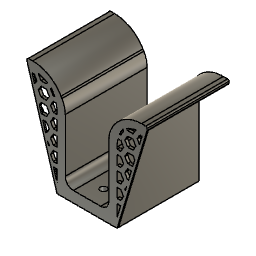
Antriebsabdeckung v4 (Autodesk Fusion 360 design; units mm, degrees)
Autodesk Fusion 360 part; units mm, degrees
note: some values were not read from the file. Set by a fixed rule: which sketch regions a step uses.
sketch "Skizze1" plane through (0, 0, 0) normal (0, 0, 1) x (1, 0, 0)
  line L0 (-250, 150) -> (-30, 150)
  line L1 (-30, 150) -> (-30, -150)
  line L2 (-30, -150) -> (-250, -150)
  line L3 (-250, -150) -> (-250, 150)
  dimension "d1" = 220
  dimension "d2" = 300
  constraint horizontal L0
  constraint vertical L1
  constraint horizontal L2
  constraint vertical L3
  measures "d1" distance of L0.start L0.end
  measures "d2" distance of L0.start L2.end
sketch "Skizze1 (2)" plane through (0, 0, 0) normal (0, 0, 1) x (1, 0, 0) in component "Component'"
  line L0 (0, 30) -> (22, 30)
  line L1 (22, 30) -> (22, 0)
  line L2 (22, 0) -> (0, 0)
  line L3 (0, 0) -> (0, 30)
  dimension "d5" = 22
  dimension "d6" = 30
  constraint horizontal L0
  constraint vertical L1
  constraint horizontal L2
  constraint vertical L3
  constraint coincident L2.end L3.start
  measures "d5" distance of L0.start L0.end
  measures "d6" distance of L0.start L2.end
extrude "Extrusion1" add sketch "Skizze1 (2)" along normal blind 4 in component "Component'"
sketch "Skizze2" plane through (0, 0, 0) normal (0, 0, 1) x (1, 0, 0) in component "Component'"
  line L0 (0, 30) -> (3, 30)
  line L1 (3, 30) -> (3, 0)
  line L2 (3, 0) -> (0, 0)
  line L3 (0, 0) -> (0, 30)
  line L4 (19, 30) -> (22, 30)
  line L5 (22, 30) -> (22, 0)
  line L6 (22, 0) -> (19, 0)
  line L7 (19, 0) -> (19, 30)
  dimension "d9" = 3
  dimension "d10" = 30
  dimension "d11" = 3
  dimension "d12" = 30
  constraint horizontal L0
  constraint vertical L1
  constraint horizontal L2
  constraint vertical L3
  constraint coincident L2.end L3.start
  constraint horizontal L4
  constraint vertical L5
  constraint horizontal L6
  constraint vertical L7
  measures "d9" distance of L0.start L0.end
  measures "d10" distance of L0.start L2.end
  measures "d11" distance of L4.start L4.end
  measures "d12" distance of L4.start L6.end
extrude "Extrusion2" add sketch "Skizze2" along normal blind 29 in component "Component'"
fillet "Abrundung1" radius 3 1 edges at (3, 15, 4) in component "Component'"
fillet "Abrundung2" radius 3 1 edges at (19, 15, 4) in component "Component'"
sketch "Skizze3" plane through (0, 0, 0) normal (0, 1, 0) x (1, 0, 0) in component "Component'"
  line L0 (22, -29) -> (27, -37.6603)
  line L1 (22, -29) -> (29, -29) construction
  line L2 (27, -37.6603) -> (24, -37.6603)
  line L3 (24, -37.6603) -> (19, -29)
  line L4 (19, -29) -> (19, -28)
  line L5 (19, -28) -> (22, -28)
  line L6 (22, -28) -> (22, -29)
  line L7 (3, -28) -> (3, -29)
  line L8 (3, -28) -> (0, -28)
  line L9 (0, -28) -> (0, -29)
  line L10 (0, -29) -> (-5, -37.6603)
  line L11 (-5, -37.6603) -> (-2, -37.6603)
  line L12 (-2, -37.6603) -> (3, -29)
  dimension "d19" = 60
  dimension "d20" = 10
  dimension "d21" = 3
  dimension "d22" = 30
  dimension "d23" = 10
  dimension "d24" = 60
  dimension "d25" = 3
  constraint horizontal L1
  constraint horizontal L2
  constraint perpendicular L2 L4
  constraint perpendicular L4 L5
  constraint perpendicular L1 L6
  constraint perpendicular L5 L7
  constraint perpendicular L7 L8
  constraint perpendicular L8 L9
  measures "d19" angle of L0 L1
  measures "d20" distance of L0.start L0.end
  measures "d21" distance of L0.end L2.end
  measures "d22" angle of L9 L10
  measures "d23" distance of L9.end L10.end
  measures "d24" angle of L10 L11
  measures "d25" distance of L10.end L11.end
extrude "Extrusion3" add sketch "Skizze3" along normal blind 30 in component "Component'"
fillet "Abrundung3" radius 12 1 edges at (22, 15, 29) in component "Component'"
fillet "Abrundung4" radius 12 1 edges at (0, 15, 29) in component "Component'"
fillet "Abrundung5" radius 9 2 edges at (19, 15, 29) (3, 15, 29) in component "Component'"
sketch "Skizze4" plane through (0, 0, 0) normal (0, 1, 0) x (1, 0, 0) in component "Component'"
  line L0 (27, -37.6603) -> (33, -37.6603)
  line L1 (33, -37.6603) -> (33, -36.1603)
  line L2 (27, -37.6603) -> (24.3973, -33.167)
  line L3 (24.3973, -33.167) -> (33, -36.1603)
  line L4 (0, -2.5) -> (22, -2.5)
  line L5 (11, -2.5) -> (11, -47.5)
  point P0 (27, -37.6603)
  dimension "d34" = 6
  dimension "d35" = 1.5
  dimension "d39" = 45
  constraint horizontal L0
  constraint coincident P0 L0.start
  constraint vertical L1
  constraint horizontal L4
  constraint vertical L5
  constraint midpoint L4 L5.start
  measures "d34" distance of P0 L0.end
  measures "d35" distance of L0.end L1.end
  measures "d39" distance of L5.start L5.end
extrude "Extrusion4" add sketch "Skizze4" along normal blind 30 in component "Component'"
fillet "Abrundung6" radius 5 1 edges at (24.4079, 15, 33.1707) in component "Component'"
fillet "Abrundung7" radius 12 1 edges at (24, 15, 37.6603) in component "Component'"
fillet "Abrundung8" radius 0.5 1 edges at (33, 15, 37.6603) in component "Component'"
fillet "Abrundung9" radius 0.5 1 edges at (33, 15, 36.1603) in component "Component'"
sketch "Skizze5" plane through (0, 0, 0) normal (0, -1, 0) x (1, 0, 0) in component "Component'"
  arc A0 (32.6643, 36.0435) -> (33, 36.5157) centre (32.5, 36.5157) ccw
  line L0 (33, 36.5157) -> (33, 37.1603)
  arc A1 (33, 37.1603) -> (32.5, 37.6603) centre (32.5, 37.1603) ccw
  line L1 (32.5, 37.6603) -> (30.9282, 37.6603)
  arc A2 (30.9282, 37.6603) -> (20.5359, 31.6603) centre (30.9282, 25.6603) ccw
  line L2 (20.5359, 31.6603) -> (20.2058, 31.0885)
  arc A3 (20.2058, 31.0885) -> (19, 26.5885) centre (28, 26.5885) ccw
  line L3 (19, 26.5885) -> (19, 7)
  arc A4 (16, 4) -> (19, 7) centre (16, 7) ccw
  line L4 (16, 4) -> (6, 4)
  arc A5 (3, 7) -> (6, 4) centre (6, 7) ccw
  line L5 (3, 7) -> (3, 26.5885)
  arc A6 (3, 26.5885) -> (1.7942, 31.0885) centre (-6, 26.5885) ccw
  line L6 (1.7942, 31.0885) -> (-2, 37.6603)
  line L7 (-2, 37.6603) -> (-5, 37.6603)
  line L8 (-5, 37.6603) -> (-1.6077, 31.7846)
  arc A7 (0, 25.7846) -> (-1.6077, 31.7846) centre (-12, 25.7846) ccw
  line L9 (0, 25.7846) -> (0, 0)
  line L10 (0, 0) -> (22, 0)
  line L11 (22, 0) -> (22, 25.7846)
  arc A8 (23.3965, 31.403) -> (22, 25.7846) centre (34, 25.7846) ccw
  arc A9 (26.1715, 33.7843) -> (23.3965, 31.403) centre (27.8146, 29.062) ccw
  line L12 (26.1715, 33.7843) -> (32.6643, 36.0435)
  line L13 (-5, 37.6603) -> (-11, 37.6603)
  line L14 (-11, 37.6603) -> (-11, 36.1603)
  line L15 (-11, 36.1603) -> (-2.3934, 33.1455)
  line L16 (-5, 37.6603) -> (-4.6132, 37.6603)
  line L17 (-4.6132, 37.6603) -> (-1.8556, 32.8839)
  line L18 (-1.8556, 32.8839) -> (-2.3934, 33.1455)
  dimension "d50" = 6
  dimension "d51" = 1.5
  constraint coincident L7.end L8.start
  constraint parallel L7 L13
  constraint perpendicular L13 L14
  constraint coincident L8 L15.end
  constraint coincident L7 L16.end
  constraint parallel L8 L17
  measures "d50" distance of L7.end L13.end
  measures "d51" distance of L13.end L14.end
extrude "Extrusion5" add sketch "Skizze5" against normal blind 30 contours L8 L13 L14 L15 in component "Component'"
fillet "Abrundung10" radius 12 1 edges at (-2, 15, 37.6603) in component "Component'"
fillet "Abrundung11" radius 0.5 1 edges at (-11, 15, 37.6603) in component "Component'"
fillet "Abrundung12" radius 0.5 1 edges at (-11, 15, 36.1603) in component "Component'"
fillet "Abrundung13" radius 5 1 edges at (-2.3934, 15, 33.1455) in component "Component'"
sketch "Skizze6" plane through (0, 0, 0) normal (0, 1, 0) x (1, 0, 0) in component "Component'"
  line L0 (0, 0) -> (22, 0)
  line L1 (11, 0) -> (11, -40)
  line L2 (0, 0) -> (-11, -36.5149)
  line L3 (0, 0) -> (-11, -36.5149)
  line L4 (-11, -36.5149) -> (-10.0425, -36.8033)
  line L5 (-10.0425, -36.8033) -> (0.9575, -0.2884)
  line L6 (0.9575, -0.2884) -> (0, 0)
  point P0 (-11, -36.5149)
  dimension "d63" = 22
  dimension "d64" = 40
  dimension "d65" = 1
  constraint coincident L0.start L2.start
  constraint horizontal L0
  constraint midpoint L0 L1.start
  constraint perpendicular L0 L1
  constraint coincident P0 L2.end
  constraint perpendicular L3 L4
  constraint parallel L3 L5
  constraint parallel L4 L6
  measures "d63" distance of L0.start L0.end
  measures "d64" distance of L1.start L1.end
  measures "d65" distance of L0.start L5.end
sketch "Skizze7" plane through (-1.5503, 0, 28.8306) normal (0, 1, 0) x (1, 0, 0) in component "Component'"
sketch "Skizze8" plane through (0, 0, 0) normal (0, 1, 0) x (1, 0, 0) in component "Component'"
sketch "Skizze9" plane through (0, 0, 0) normal (0, 1, 0) x (1, 0, 0) in component "Component'"
  line L0 (0, 0) -> (22, 0)
  line L1 (22, 0) -> (33, -36.5157)
  line L2 (22, 0) -> (33, -36.5157)
  line L3 (33, -36.5157) -> (32.0425, -36.8041)
  line L4 (32.0425, -36.8041) -> (21.0425, -0.2884)
  line L5 (21.0425, -0.2884) -> (22, 0)
  point P0 (33, -36.5157)
  dimension "d98" = 22
  dimension "d99" = 1
  constraint coincident L0.start origin
  constraint horizontal L0
  constraint coincident P0 L1.end
  constraint perpendicular L2 L3
  constraint parallel L2 L4
  constraint parallel L3 L5
  constraint parallel L1 L2
  measures "d98" distance of L0.start L0.end
  measures "d99" distance of L0.end L4.end
extrude "Extrusion6" add sketch "Skizze9" sketch "Skizze6" along normal blind 1 of sketch 2 in component "Component'"
fillet "Abrundung14" radius 0.5 1 edges at (-4.8565, 1, 19.5882) in component "Component'"
fillet "Abrundung15" radius 0.5 1 edges at (-5.4584, 1, 18.1194) in component "Component'"
fillet "Abrundung16" radius 0.5 1 edges at (27.4584, 1, 18.1198) in component "Component'"
fillet "Abrundung17" radius 0.5 1 edges at (26.8569, 1, 19.5898) in component "Component'"
sketch "Skizze10" plane through (0, 0, 0) normal (0, 1, 0) x (1, 0, 0) in component "Component'"
  line L0 (-1.3615, -7.8038) -> (0.6385, -7.804)
  line L1 (0.6389, -4.3399) -> (-0.6992, -4.3399)
  line L2 (-1.6032, -7.3682) -> (-1.3615, -7.8038)
  line L3 (-1.3615, -7.8038) -> (-0.3615, -7.8039) construction
  line L4 (-2.3613, -11.2682) -> (-1.3615, -9.536)
  line L5 (-1.3615, -9.536) -> (-0.3615, -9.5359) construction
  line L6 (-1.3615, -9.536) -> (0.6385, -9.5358)
  line L7 (-1.3611, -13.0001) -> (-2.3613, -11.2682)
  line L8 (0.6389, -12.9999) -> (-1.3611, -13.0001)
  line L9 (-1.3615, -9.536) -> (-0.3615, -9.5359) construction
  line L10 (-2.3613, -11.2682) -> (-1.3615, -9.536)
  line L11 (-1.3615, -9.536) -> (0.6385, -9.5358)
  line L12 (-1.3611, -13.0001) -> (-2.3613, -11.2682)
  line L13 (0.6389, -12.9999) -> (-1.3611, -13.0001)
  line L14 (-1.3613, -33.7846) -> (-3.4883, -33.7846) construction
  line L15 (-1.3613, -30.3205) -> (-2.3613, -32.0526)
  line L16 (-2.3613, -32.0526) -> (-1.3613, -33.7846)
  line L17 (0.6387, -30.3205) -> (-1.3613, -30.3205)
  line L18 (-7.3878, -32.0984) -> (-8.5461, -30.1296)
  line L19 (-9.6744, -33.7729) -> (-8.3545, -33.7729)
  line L20 (-8.3545, -33.7729) -> (-7.3878, -32.0984)
  line L21 (-1.3613, -18.1962) -> (0.6387, -18.1962)
  line L22 (-1.3613, -14.7321) -> (-2.3613, -16.4641)
  line L23 (-2.3613, -16.4641) -> (-1.3613, -18.1962)
  line L24 (0.6387, -14.7321) -> (-1.3613, -14.7321)
  line L25 (-1.3613, -28.5885) -> (0.6387, -28.5885)
  line L26 (-1.3613, -25.1244) -> (-2.3613, -26.8564)
  line L27 (-2.3613, -26.8564) -> (-1.3613, -28.5885)
  line L28 (0.6387, -25.1244) -> (-1.3613, -25.1244)
  line L29 (-2.8613, -34.6506) -> (-3.8613, -32.9186)
  line L30 (-5.8613, -32.9186) -> (-6.8613, -34.6506)
  line L31 (-6.8613, -34.6506) -> (-5.8613, -36.3827)
  line L32 (-3.8613, -32.9186) -> (-5.8613, -32.9186)
  line L33 (-2.8613, -29.4545) -> (-3.8613, -27.7224)
  line L34 (-5.8613, -31.1865) -> (-3.8613, -31.1865)
  line L35 (-5.8613, -27.7224) -> (-6.8613, -29.4545)
  line L36 (-3.8613, -31.1865) -> (-2.8613, -29.4545)
  line L37 (-6.8613, -29.4545) -> (-5.8613, -31.1865)
  line L38 (-3.8613, -27.7224) -> (-5.8613, -27.7224)
  line L39 (-2.8613, -19.0622) -> (-3.8684, -17.3179)
  line L40 (-5.6515, -20.7821) -> (-3.8543, -20.7821)
  line L41 (-3.8543, -20.7821) -> (-2.8613, -19.0622)
  line L42 (-3.8684, -17.3179) -> (-4.5785, -17.3174)
  line L43 (-1.3613, -23.3923) -> (0.6387, -23.3923)
  line L44 (-1.3613, -19.9282) -> (-2.3613, -21.6603)
  line L45 (-2.3613, -21.6603) -> (-1.3613, -23.3923)
  line L46 (0.6387, -19.9282) -> (-1.3613, -19.9282)
  line L47 (0, 0) -> (22, 0)
  line L48 (11, 0) -> (11, -45)
  line L49 (1.1387, -3.4737) -> (-0.4406, -3.4736)
  line L50 (22, -3.467) -> (22, -25.7846)
  line L51 (0.6387, -25.1244) -> (0.6387, -28.5885)
  line L52 (0.6387, -23.3923) -> (0.6387, -19.9282)
  line L53 (0.6387, -14.7321) -> (0.6387, -18.1962)
  line L54 (0.6387, -30.3205) -> (-1.3613, -33.7846)
  line L55 (-2.8613, -34.6506) -> (-5.8613, -36.3827)
  line L56 (0.6389, -4.3399) -> (0.6385, -7.804)
  line L57 (1.1387, -3.4737) -> (1.1387, -8.6699)
  line L58 (0.6385, -9.5358) -> (0.6389, -12.9999)
  line L59 (1.1387, -8.6699) -> (1.1387, -13.866)
  line L60 (1.1387, -13.866) -> (1.1387, -19.0622)
  line L61 (1.1387, -19.0622) -> (1.1387, -24.2583)
  line L62 (1.1387, -24.2583) -> (1.1387, -29.4545)
  line L63 (1.1387, -29.4545) -> (0.6387, -31.9352)
  line L64 (0.6387, -31.9352) -> (-0.8065, -33.9794)
  line L65 (-0.8065, -33.9794) -> (-1.8613, -34.6506)
  line L66 (-6.4159, -37.1736) -> (-1.8613, -34.6506)
  line L67 (-5.8613, -25.9904) -> (-3.8613, -25.9904)
  line L68 (-3.8613, -22.5263) -> (-5.8613, -22.5263)
  line L69 (-6.8613, -24.2583) -> (-5.8613, -25.9904)
  line L70 (-5.8613, -22.5263) -> (-6.8613, -24.2583)
  line L71 (-2.8613, -24.2583) -> (-3.8613, -22.5263)
  line L72 (-3.8613, -25.9904) -> (-2.8613, -24.2583)
  line L73 (-2.8613, -13.866) -> (-3.3053, -13.07)
  line L74 (-3.8613, -15.5981) -> (-2.8613, -13.866)
  line L75 (-4.06, -15.5981) -> (-3.8613, -15.5981)
  line L76 (-10.3496, -35.9533) -> (-8.3613, -35.5167)
  line L77 (-8.3613, -35.5167) -> (-7.3613, -37.2487)
  line L78 (-6.4159, -37.1736) -> (-7.3613, -37.2487)
  line L79 (-10.3496, -35.9533) -> (-4.4333, -16.8484)
  line L80 (-4.4333, -16.8484) -> (-0.4406, -3.4736)
  line L81 (-1.6032, -7.3682) -> (-1.9229, -8.4393)
  line L82 (-0.4406, -3.4736) -> (-0.6992, -4.3399)
  line L83 (-1.6032, -7.3682) -> (-1.9229, -8.4393)
  line L84 (-5.6515, -20.7821) -> (-7.4138, -26.5466)
  line L85 (27.8613, -22.5263) -> (28.8613, -24.2583)
  line L86 (21.3611, -12.9999) -> (23.3611, -13.0001)
  line L87 (23.3611, -13.0001) -> (24.3613, -11.2682)
  line L88 (25.8613, -15.5981) -> (24.8613, -13.866)
  line L89 (20.8613, -13.866) -> (20.8613, -19.0622)
  line L90 (24.8613, -13.866) -> (25.3053, -13.07)
  line L91 (23.3611, -13.0001) -> (24.3613, -11.2682)
  line L92 (20.8613, -3.4737) -> (22.4406, -3.4736)
  line L93 (24.3613, -16.4641) -> (23.3613, -18.1962)
  line L94 (23.3613, -14.7321) -> (24.3613, -16.4641)
  line L95 (23.3615, -9.536) -> (21.3615, -9.5358)
  line L96 (21.3611, -12.9999) -> (23.3611, -13.0001)
  line L97 (21.3613, -14.7321) -> (21.3613, -18.1962)
  line L98 (23.6032, -7.3682) -> (23.3615, -7.8038)
  line L99 (21.3613, -14.7321) -> (23.3613, -14.7321)
  line L100 (22.4406, -3.4736) -> (22.6992, -4.3399)
  line L101 (26.06, -15.5981) -> (25.8613, -15.5981)
  line L102 (20.8613, -3.4737) -> (20.8613, -8.6699)
  line L103 (31.6744, -33.7729) -> (30.3545, -33.7729)
  line L104 (23.3613, -30.3205) -> (24.3613, -32.0526)
  line L105 (29.3878, -32.0984) -> (30.5461, -30.1296)
  line L106 (21.3613, -31.9352) -> (22.8065, -33.9794)
  line L107 (21.3613, -30.3205) -> (23.3613, -30.3205)
  line L108 (27.8613, -31.1865) -> (25.8613, -31.1865)
  line L109 (28.8613, -24.2583) -> (27.8613, -25.9904)
  line L110 (25.8684, -17.3179) -> (26.5785, -17.3174)
  line L111 (27.8613, -32.9186) -> (28.8613, -34.6506)
  line L112 (21.3613, -25.1244) -> (21.3613, -28.5885)
  line L113 (30.3545, -33.7729) -> (29.3878, -32.0984)
  line L114 (27.6515, -20.7821) -> (25.8543, -20.7821)
  line L115 (25.8613, -27.7224) -> (27.8613, -27.7224)
  line L116 (24.3613, -26.8564) -> (23.3613, -28.5885)
  line L117 (21.3613, -30.3205) -> (23.3613, -33.7846)
  line L118 (25.8613, -32.9186) -> (27.8613, -32.9186)
  line L119 (20.8613, -24.2583) -> (20.8613, -29.4545)
  line L120 (25.8613, -22.5263) -> (27.8613, -22.5263)
  line L121 (28.8613, -29.4545) -> (27.8613, -31.1865)
  line L122 (27.8613, -27.7224) -> (28.8613, -29.4545)
  line L123 (23.3613, -28.5885) -> (21.3613, -28.5885)
  line L124 (24.3613, -32.0526) -> (23.3613, -33.7846)
  line L125 (28.4159, -37.1736) -> (29.3613, -37.2487)
  line L126 (24.8613, -29.4545) -> (25.8613, -27.7224)
  line L127 (25.8543, -20.7821) -> (24.8613, -19.0622)
  line L128 (20.8613, -29.4545) -> (21.3613, -31.9352)
  line L129 (23.3613, -23.3923) -> (21.3613, -23.3923)
  line L130 (24.8613, -19.0622) -> (25.8684, -17.3179)
  line L131 (25.8613, -25.9904) -> (24.8613, -24.2583)
  line L132 (23.3613, -18.1962) -> (21.3613, -18.1962)
  line L133 (23.3613, -25.1244) -> (24.3613, -26.8564)
  line L134 (27.6515, -20.7821) -> (29.4138, -26.5466)
  line L135 (30.3613, -35.5167) -> (29.3613, -37.2487)
  line L136 (23.3613, -33.7846) -> (25.4883, -33.7846) construction
  line L137 (24.8613, -34.6506) -> (25.8613, -32.9186)
  line L138 (22.8065, -33.9794) -> (23.8613, -34.6506)
  line L139 (24.3613, -21.6603) -> (23.3613, -23.3923)
  line L140 (20.8613, -19.0622) -> (20.8613, -24.2583)
  line L141 (21.3613, -23.3923) -> (21.3613, -19.9282)
  line L142 (27.8613, -25.9904) -> (25.8613, -25.9904)
  line L143 (24.8613, -24.2583) -> (25.8613, -22.5263)
  line L144 (32.3496, -35.9533) -> (30.3613, -35.5167)
  line L145 (28.4159, -37.1736) -> (23.8613, -34.6506)
  line L146 (26.4333, -16.8484) -> (22.4406, -3.4736)
  line L147 (21.3613, -19.9282) -> (23.3613, -19.9282)
  line L148 (21.3615, -9.5358) -> (21.3611, -12.9999)
  line L149 (24.8613, -34.6506) -> (27.8613, -36.3827)
  line L150 (21.3613, -25.1244) -> (23.3613, -25.1244)
  line L151 (28.8613, -34.6506) -> (27.8613, -36.3827)
  line L152 (25.8613, -31.1865) -> (24.8613, -29.4545)
  line L153 (24.3613, -11.2682) -> (23.3615, -9.536)
  line L154 (23.3613, -19.9282) -> (24.3613, -21.6603)
  line L155 (23.3615, -9.536) -> (22.3615, -9.5359) construction
  line L156 (23.3615, -9.536) -> (21.3615, -9.5358)
  line L157 (24.3613, -11.2682) -> (23.3615, -9.536)
  line L158 (23.6032, -7.3682) -> (23.9229, -8.4393)
  line L159 (23.3615, -7.8038) -> (21.3615, -7.804)
  line L160 (32.3496, -35.9533) -> (26.4333, -16.8484)
  line L161 (21.3611, -4.3399) -> (21.3615, -7.804)
  line L162 (21.3611, -4.3399) -> (22.6992, -4.3399)
  line L163 (23.3615, -7.8038) -> (22.3615, -7.8039) construction
  line L164 (23.6032, -7.3682) -> (23.9229, -8.4393)
  line L165 (20.8613, -8.6699) -> (20.8613, -13.866)
  line L166 (23.3615, -9.536) -> (22.3615, -9.5359) construction
  point P0 (1.1387, -8.6699)
  point P1 (-0.3613, -11.268)
  point P2 (-0.3613, -21.6603)
  point P3 (-4.8613, -19.0622)
  point P4 (-0.3613, -26.8564)
  point P5 (-4.8613, -29.4545)
  point P6 (-4.66, -23.9097)
  point P7 (-9.3613, -32.0526)
  point P8 (-4.8613, -34.6506)
  point P9 (-0.3613, -32.0526)
  point P10 (-9.3613, -37.2487)
  point P11 (-9.3613, -37.2487)
  point P12 (-0.3613, -32.0526)
  point P13 (-9.3613, -32.0526)
  point P14 (-0.3613, -16.4641)
  point P15 (-4.8613, -13.866)
  point P16 (-0.3613, -26.8564)
  point P17 (-4.8613, -34.6506)
  point P18 (-4.8613, -29.4545)
  point P19 (-4.66, -23.9097)
  point P20 (-4.8613, -19.0622)
  point P21 (-0.3613, -21.6603)
  point P22 (-4.8613, -24.2583)
  point P23 (-4.8613, -24.2583)
  point P24 (-4.8613, -13.866)
  point P25 (-4.8613, -13.866)
  point P26 (22.3613, -21.6603)
  point P27 (26.8613, -19.0622)
  point P28 (26.8613, -13.866)
  point P29 (26.8613, -19.0622)
  point P30 (20.8613, -8.6699)
  point P31 (26.8613, -13.866)
  point P32 (26.8613, -24.2583)
  point P33 (22.3613, -21.6603)
  point P34 (26.8613, -24.2583)
  point P35 (26.66, -23.9097)
  point P36 (26.66, -23.9097)
  point P37 (22.3613, -16.4641)
  point P38 (26.8613, -13.866)
  point P39 (22.3613, -26.8564)
  point P40 (26.8613, -34.6506)
  point P41 (26.8613, -29.4545)
  point P42 (22.3613, -32.0526)
  point P43 (22.3613, -11.268)
  point P44 (26.8613, -29.4545)
  point P45 (22.3613, -32.0526)
  point P46 (31.3613, -37.2487)
  point P47 (22.3613, -26.8564)
  point P48 (31.3613, -32.0526)
  point P49 (31.3613, -32.0526)
  point P50 (31.3613, -37.2487)
  point P51 (26.8613, -34.6506)
  dimension "d119" = 0
  dimension "d144" = 22
  dimension "d145" = 45
  dimension "d149" = 20
  constraint horizontal L14
  constraint coincident P11 P10
  constraint coincident P13 P7
  constraint coincident P17 P8
  constraint coincident P18 P5
  constraint coincident P19 P6
  constraint coincident P21 P2
  constraint coincident P12 P9
  constraint coincident P16 P4
  constraint coincident P20 P3
  constraint coincident L47.start origin
  constraint horizontal L47
  constraint vertical L48
  constraint midpoint L47 L48.start
  constraint perpendicular L25 L51
  constraint perpendicular L46 L52
  constraint perpendicular L31 L55
  constraint coincident P0 L57.end
  constraint coincident P23 P22
  constraint coincident P25 P24
  constraint coincident L1.end L80
  constraint horizontal L1
  constraint coincident L2.start L80
  constraint coincident L81.end L80
  constraint coincident L73.end L80
  constraint coincident L75.start L80
  constraint coincident L42.end L79
  constraint coincident L40.start L79
  constraint horizontal L40
  constraint horizontal L19
  constraint coincident L19.start L79
  constraint coincident L18.end L79
  constraint symmetric L49.start L48 L92.start
  constraint symmetric L81.end L48 L158.end
  constraint symmetric L0.start L48 L98.end
  constraint symmetric L0.end L48 L159.end
  constraint symmetric L1.start L48 L161.start
  constraint symmetric L1.end L48 L100.end
  constraint symmetric L2.start L48 L98.start
  constraint symmetric L3.end L48 L163.end
  constraint symmetric L7.start L48 L86.end
  constraint symmetric L4.start L48 L87.end
  constraint symmetric P0 L48 P30
  constraint symmetric L5.end L48 L155.end
  constraint symmetric L59.end L48 L89.start
  constraint symmetric L6.end L48 L95.end
  constraint symmetric L4.end L48 L95.start
  constraint symmetric L8.start L48 L86.start
  constraint symmetric P1 L48 P43
  constraint symmetric L60.end L48 L89.end
  constraint symmetric L61.end L48 L119.start
  constraint symmetric P21 L48 P33
  constraint symmetric P20 L48 P29
  constraint symmetric L62.end L48 L119.end
  constraint symmetric P16 L48 P47
  constraint symmetric P18 L48 P44
  constraint symmetric P19 L48 P36
  constraint symmetric P13 L48 P49
  constraint symmetric L65.end L48 L138.end
  constraint symmetric P17 L48 P51
  constraint symmetric P12 L48 P45
  constraint symmetric L66.start L48 L125.start
  constraint symmetric P11 L48 P50
  constraint symmetric L14.start L48 L117.end
  constraint symmetric L15.end L48 L104.end
  constraint symmetric L17.start L48 L107.start
  constraint symmetric L15.start L48 L104.start
  constraint symmetric L14.end L48 L136.end
  constraint symmetric L19.start L48 L103.start
  constraint symmetric L19.end L48 L103.end
  constraint symmetric L18.end L48 L105.end
  constraint symmetric L18.start L48 L105.start
  constraint symmetric L21.start L48 L93.end
  constraint symmetric L22.end L48 L93.start
  constraint symmetric L21.end L48 L97.end
  constraint symmetric L24.start L48 L97.start
  constraint symmetric P14 L48 P37
  constraint symmetric L22.start L48 L94.start
  constraint symmetric P25 L48 P38
  constraint symmetric L25.start L48 L116.end
  constraint symmetric L26.end L48 L116.start
  constraint symmetric L25.end L48 L112.end
  constraint symmetric L28.start L48 L112.start
  constraint symmetric L26.start L48 L133.start
  constraint symmetric L31.end L48 L149.end
  constraint symmetric L30.end L48 L111.end
  constraint symmetric L29.end L48 L118.start
  constraint symmetric L29.start L48 L137.start
  constraint symmetric L30.start L48 L111.start
  constraint symmetric L34.start L48 L108.start
  constraint symmetric L35.end L48 L121.start
  constraint symmetric L34.end L48 L108.end
  constraint symmetric L33.end L48 L115.start
  constraint symmetric L33.start L48 L126.start
  constraint symmetric L35.start L48 L115.end
  constraint symmetric L40.start L48 L114.start
  constraint symmetric L40.end L48 L114.end
  constraint symmetric L39.end L48 L110.start
  constraint symmetric L39.start L48 L127.end
  constraint symmetric L42.end L48 L110.end
  constraint symmetric L43.start L48 L129.start
  constraint symmetric L44.end L48 L139.start
  constraint symmetric L43.end L48 L129.end
  constraint symmetric L46.start L48 L141.end
  constraint symmetric L44.start L48 L147.end
  constraint symmetric L48 L49.end L92.end
  constraint symmetric L48 P0 P30
  constraint symmetric L48 L63.end L106.start
  constraint symmetric L48 L64.end L106.end
  constraint symmetric L48 P23 P34
  constraint symmetric L48 L68.end L85.start
  constraint symmetric L48 L67.start L109.end
  constraint symmetric L48 L69.start L85.end
  constraint symmetric L48 L68.start L120.start
  constraint symmetric L48 L67.end L131.start
  constraint symmetric L48 L71.start L131.end
  constraint symmetric L48 P25 P38
  constraint symmetric L48 L75.start L101.start
  constraint symmetric L48 L73.end L90.end
  constraint symmetric L48 L74.start L88.start
  constraint symmetric L48 L73.start L88.end
  constraint symmetric L48 L77.end L125.end
  constraint symmetric L48 L76.start L144.start
  constraint symmetric L48 L76.end L135.start
  constraint symmetric L48 L79.end L146.start
  constraint symmetric L48 L84.end L134.end
  measures "d119" angle of L0 L3
  measures "d144" distance of L47.start L47.end
  measures "d145" distance of L48.start L48.end
  measures "d149" distance of L76.start L79.end
extrude "Extrusion7" add sketch "Skizze10" along normal blind 1 contours L0 L1 L2 L18 L19 L20 L39 L40 L41 L42 L49 L56 L57 L59 L60 L61 L62 L63 L64 L65 L66 L67 L68 L69 L70 L71 L72 L73 L74 L75 L76 L77 L78 L79 L80 L81 L82 L83 L84 | L50 L85 L88 L89 L90 L92 L98 L101 L102 L103 L105 L106 L109 L110 L113 L114 L119 L120 L125 L127 L128 L130 L131 L134 L135 L138 L140 L142 L143 L144 L145 L146 L158 L159 L160 L161 L162 L164 L165 in component "Component'"
sketch "Skizze2 (2)" plane through (0, 0, 0) normal (0, 0, 1) x (1, 0, 0)
  line L0 (0, 0) -> (22, 0)
  line L1 (11, 0) -> (11, 6)
  line L2 (11, 6) -> (11, 24)
  line L3 (11, 24) -> (11, 30)
  circle A0 centre (11, 24) radius 1.2
  circle A1 centre (11, 6) radius 1.2
  dimension "d152" = 22
  dimension "d153" = 6
  dimension "d154" = 18
  dimension "d156" = 6
  dimension "d157" = 2.4
  dimension "d158" = 2.4
  constraint horizontal L0
  constraint vertical L1
  constraint midpoint L0 L1.start
  constraint vertical L2
  constraint parallel L2 L3
  constraint coincident L2.end L3.start
  constraint coincident L1.end L2.start
  constraint coincident L0.start origin
  measures "d152" distance of L0.start L0.end
  measures "d153" distance of L1.start L1.end
  measures "d154" distance of L1.end L2.end
  measures "d156" distance of L2.end L3.end
  measures "d157" diameter of A0
  measures "d158" diameter of A1
extrude "Extrusion8" cut sketch "Skizze2 (2)" along normal blind 4 in component "Component'"
component "Component" placed x (1, 0, 0) y (0, 1, 0) z (0, 0, 1) at (0, 0, 0)
component "Component'" placed x (1, 0, 0) y (0, 1, 0) z (0, 0, 1) at (0, 0, 0) in component "Component"
